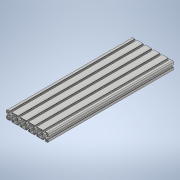
# Autodesk Inventor part: 20100 dai 300
Saved by Autodesk Inventor 2020 (Build 240168000, 168)
## iProperties
Created: 2020-04-28
Part Number: 20100 dai 300
Material: Generic
Document SubType Name: Modeling
Designer: Dell-T1700
Density: 1 g/cm^3
Appearance: Default
Author: Dell-T1700
Autodesk Inventor part; units mm, degrees
ref_plane "YZ Plane" through (0, 0, 0) normal (1, 0, 0) x (0, 1, 0)
ref_plane "XZ Plane" through (0, 0, 0) normal (0, 1, 0) x (-1, 0, 0)
ref_plane "XY Plane" through (0, 0, 0) normal (0, 0, 1) x (1, 0, 0)
sketch "Sketch1" plane through (0, 0, 0) normal (0, 0, 1) x (1, 0, 0)
  line L0 (-2.55, -10) -> (-2.55, -9.25)
  line L1 (-2.55, -9.25) -> (-2.05, -9.25)
  line L2 (-7.75, -10) -> (-2.55, -10)
  line L3 (-2.05, -9.25) -> (-2.05, -7)
  line L4 (-2.05, -7) -> (-3.05, -7)
  line L5 (-3.05, -9.1) -> (-3.05, -7)
  line L6 (-3.05, -9.1) -> (-5.125, -9.1)
  line L7 (-5.125, -9.1) -> (-5.125, -5.8321)
  line L8 (-8, -9.25) -> (-5.775, -9.25)
  line L9 (-5.775, -9.25) -> (-5.775, -5.775)
  line L10 (-2.2929, -3) -> (2.2929, -3)
  line L11 (3, -2.2929) -> (3, 2.2929)
  line L12 (2.2929, 3) -> (-2.2929, 3)
  line L13 (-3, 2.2929) -> (-3, -2.2929)
  line L14 (-2.2929, -3) -> (-5.125, -5.8321)
  line L15 (-3, -2.2929) -> (-5.8321, -5.125)
  line L16 (-9.1, -5.125) -> (-5.8321, -5.125)
  line L17 (-9.25, -5.775) -> (-5.775, -5.775)
  line L18 (-9.25, -8) -> (-9.25, -5.775)
  line L19 (-10, -7.75) -> (-10, -2.55)
  line L20 (-9.1, -3.05) -> (-9.1, -5.125)
  line L21 (-9.1, -3.05) -> (-7, -3.05)
  line L22 (-9.25, -2.55) -> (-9.25, -2.05)
  line L23 (-9.25, -2.05) -> (-7, -2.05)
  line L24 (-7, -2.05) -> (-7, -3.05)
  line L25 (-10, -2.55) -> (-9.25, -2.55)
  arc A0 (-9.25, -8) -> (-8, -9.25) centre (-8, -8) ccw
  arc A1 (-10, -7.75) -> (-7.75, -10) centre (-7.75, -7.75) ccw
  line L26 (3, -2.2929) -> (5.8321, -5.125)
  line L27 (2.2929, -3) -> (5.125, -5.8321)
  line L28 (5.775, -9.25) -> (5.775, -5.775)
  line L29 (8, -9.25) -> (5.775, -9.25)
  line L30 (7.75, -10) -> (2.55, -10)
  line L31 (3.05, -9.1) -> (5.125, -9.1)
  line L32 (2.55, -10) -> (2.55, -9.25)
  line L33 (3.05, -9.1) -> (3.05, -7)
  line L34 (2.05, -9.25) -> (2.05, -7)
  line L35 (2.55, -9.25) -> (2.05, -9.25)
  line L36 (2.05, -7) -> (3.05, -7)
  line L37 (5.125, -9.1) -> (5.125, -5.8321)
  arc A2 (8, -9.25) -> (9.25, -8) centre (8, -8) ccw
  arc A3 (7.75, -10) -> (10, -7.75) centre (7.75, -7.75) ccw
  line L38 (9.25, -8) -> (9.25, -5.775)
  line L39 (10, -7.75) -> (10, -2.55)
  line L40 (9.25, -5.775) -> (5.775, -5.775)
  line L41 (9.1, -5.125) -> (5.8321, -5.125)
  line L42 (9.1, -3.05) -> (7, -3.05)
  line L43 (7, -2.05) -> (7, -3.05)
  line L44 (9.25, -2.05) -> (7, -2.05)
  line L45 (9.25, -2.55) -> (9.25, -2.05)
  line L46 (10, -2.55) -> (9.25, -2.55)
  line L47 (9.1, -3.05) -> (9.1, -5.125)
  line L48 (2.2929, 3) -> (5.125, 5.8321)
  line L49 (3, 2.2929) -> (5.8321, 5.125)
  line L50 (9.25, 5.775) -> (5.775, 5.775)
  line L51 (9.25, 8) -> (9.25, 5.775)
  line L52 (10, 7.75) -> (10, 2.55)
  line L53 (9.1, 3.05) -> (9.1, 5.125)
  line L54 (10, 2.55) -> (9.25, 2.55)
  line L55 (9.1, 3.05) -> (7, 3.05)
  line L56 (9.25, 2.05) -> (7, 2.05)
  line L57 (9.25, 2.55) -> (9.25, 2.05)
  line L58 (7, 2.05) -> (7, 3.05)
  line L59 (9.1, 5.125) -> (5.8321, 5.125)
  arc A4 (9.25, 8) -> (8, 9.25) centre (8, 8) ccw
  arc A5 (10, 7.75) -> (7.75, 10) centre (7.75, 7.75) ccw
  line L60 (8, 9.25) -> (5.775, 9.25)
  line L61 (7.75, 10) -> (2.55, 10)
  line L62 (5.775, 9.25) -> (5.775, 5.775)
  line L63 (5.125, 9.1) -> (5.125, 5.8321)
  line L64 (3.05, 9.1) -> (3.05, 7)
  line L65 (2.05, 7) -> (3.05, 7)
  line L66 (2.05, 9.25) -> (2.05, 7)
  line L67 (2.55, 9.25) -> (2.05, 9.25)
  line L68 (2.55, 10) -> (2.55, 9.25)
  line L69 (3.05, 9.1) -> (5.125, 9.1)
  line L70 (-3, 2.2929) -> (-5.8321, 5.125)
  line L71 (-2.2929, 3) -> (-5.125, 5.8321)
  line L72 (-5.775, 9.25) -> (-5.775, 5.775)
  line L73 (-8, 9.25) -> (-5.775, 9.25)
  line L74 (-7.75, 10) -> (-2.55, 10)
  line L75 (-3.05, 9.1) -> (-5.125, 9.1)
  line L76 (-2.55, 10) -> (-2.55, 9.25)
  line L77 (-3.05, 9.1) -> (-3.05, 7)
  line L78 (-2.05, 9.25) -> (-2.05, 7)
  line L79 (-2.55, 9.25) -> (-2.05, 9.25)
  line L80 (-2.05, 7) -> (-3.05, 7)
  line L81 (-5.125, 9.1) -> (-5.125, 5.8321)
  arc A6 (-8, 9.25) -> (-9.25, 8) centre (-8, 8) ccw
  arc A7 (-7.75, 10) -> (-10, 7.75) centre (-7.75, 7.75) ccw
  line L82 (-9.25, 8) -> (-9.25, 5.775)
  line L83 (-10, 7.75) -> (-10, 2.55)
  line L84 (-9.25, 5.775) -> (-5.775, 5.775)
  line L85 (-9.1, 5.125) -> (-5.8321, 5.125)
  line L86 (-9.1, 3.05) -> (-7, 3.05)
  line L87 (-7, 2.05) -> (-7, 3.05)
  line L88 (-9.25, 2.05) -> (-7, 2.05)
  line L89 (-9.25, 2.55) -> (-9.25, 2.05)
  line L90 (-10, 2.55) -> (-9.25, 2.55)
  line L91 (-9.1, 3.05) -> (-9.1, 5.125)
  circle A8 centre (0, 0) radius 2
  line L92 (17.45, -10) -> (17.45, -9.25)
  line L93 (17.45, -9.25) -> (17.95, -9.25)
  line L94 (12.25, -10) -> (17.45, -10)
  line L95 (17.95, -9.25) -> (17.95, -7)
  line L96 (17.95, -7) -> (16.95, -7)
  line L97 (17, -2.2929) -> (14.1679, -5.125)
  line L98 (17.7071, -3) -> (14.875, -5.8321)
  line L99 (14.225, -9.25) -> (14.225, -5.775)
  line L100 (14.875, -9.1) -> (14.875, -5.8321)
  line L101 (16.95, -9.1) -> (16.95, -7)
  line L102 (16.95, -9.1) -> (14.875, -9.1)
  line L103 (12, -9.25) -> (14.225, -9.25)
  line L104 (10.75, -5.775) -> (14.225, -5.775)
  line L105 (10.9, -5.125) -> (14.1679, -5.125)
  line L106 (10.75, -8) -> (10.75, -5.775)
  line L107 (10, -7.75) -> (10, -2.55)
  line L108 (10.9, -3.05) -> (10.9, -5.125)
  line L109 (13, -2.05) -> (13, -3.05)
  line L110 (10.9, -3.05) -> (13, -3.05)
  line L111 (10.75, -2.05) -> (13, -2.05)
  line L112 (10.75, -2.55) -> (10.75, -2.05)
  line L113 (10, -2.55) -> (10.75, -2.55)
  arc A9 (10, -7.75) -> (12.25, -10) centre (12.25, -7.75) ccw
  arc A10 (10.75, -8) -> (12, -9.25) centre (12, -8) ccw
  line L114 (23, -2.2929) -> (25.8321, -5.125)
  line L115 (22.2929, -3) -> (25.125, -5.8321)
  line L116 (22.05, -9.25) -> (22.05, -7)
  line L117 (22.55, -10) -> (22.55, -9.25)
  line L118 (22.55, -9.25) -> (22.05, -9.25)
  line L119 (22.05, -7) -> (23.05, -7)
  line L120 (23.05, -9.1) -> (23.05, -7)
  line L121 (23.05, -9.1) -> (25.125, -9.1)
  line L122 (27.75, -10) -> (22.55, -10)
  line L123 (27, -2.05) -> (27, -3.05)
  line L124 (25.125, -9.1) -> (25.125, -5.8321)
  line L125 (29.1, -5.125) -> (25.8321, -5.125)
  line L126 (29.1, -3.05) -> (27, -3.05)
  line L127 (29.1, -3.05) -> (29.1, -5.125)
  line L128 (29.25, -2.05) -> (27, -2.05)
  line L129 (29.25, -2.55) -> (29.25, -2.05)
  line L130 (30, -2.55) -> (29.25, -2.55)
  line L131 (30, -7.75) -> (30, -2.55)
  line L132 (25.775, -9.25) -> (25.775, -5.775)
  line L133 (29.25, -5.775) -> (25.775, -5.775)
  line L134 (28, -9.25) -> (25.775, -9.25)
  line L135 (29.25, -8) -> (29.25, -5.775)
  arc A11 (28, -9.25) -> (29.25, -8) centre (28, -8) ccw
  arc A12 (27.75, -10) -> (30, -7.75) centre (27.75, -7.75) ccw
  arc A13 (29.25, 8) -> (28, 9.25) centre (28, 8) ccw
  arc A14 (30, 7.75) -> (27.75, 10) centre (27.75, 7.75) ccw
  line L136 (29.25, 2.05) -> (27, 2.05)
  line L137 (29.25, 2.55) -> (29.25, 2.05)
  line L138 (30, 2.55) -> (29.25, 2.55)
  line L139 (27, 2.05) -> (27, 3.05)
  line L140 (29.1, 3.05) -> (27, 3.05)
  line L141 (29.1, 3.05) -> (29.1, 5.125)
  line L142 (29.1, 5.125) -> (25.8321, 5.125)
  line L143 (23, 2.2929) -> (25.8321, 5.125)
  line L144 (22.2929, 3) -> (25.125, 5.8321)
  line L145 (30, 7.75) -> (30, 2.55)
  line L146 (29.25, 5.775) -> (25.775, 5.775)
  line L147 (29.25, 8) -> (29.25, 5.775)
  line L148 (28, 9.25) -> (25.775, 9.25)
  line L149 (25.775, 9.25) -> (25.775, 5.775)
  line L150 (25.125, 9.1) -> (25.125, 5.8321)
  line L151 (27.75, 10) -> (22.55, 10)
  line L152 (23.05, 9.1) -> (25.125, 9.1)
  line L153 (22.55, 10) -> (22.55, 9.25)
  line L154 (23.05, 9.1) -> (23.05, 7)
  line L155 (22.05, 7) -> (23.05, 7)
  line L156 (22.05, 9.25) -> (22.05, 7)
  line L157 (22.55, 9.25) -> (22.05, 9.25)
  line L158 (17.95, 9.25) -> (17.95, 7)
  line L159 (17.45, 9.25) -> (17.95, 9.25)
  line L160 (17.95, 7) -> (16.95, 7)
  line L161 (16.95, 9.1) -> (16.95, 7)
  line L162 (14.225, 9.25) -> (14.225, 5.775)
  line L163 (12, 9.25) -> (14.225, 9.25)
  line L164 (10.9, 5.125) -> (14.1679, 5.125)
  line L165 (10.75, 5.775) -> (14.225, 5.775)
  line L166 (10.75, 8) -> (10.75, 5.775)
  arc A15 (12, 9.25) -> (10.75, 8) centre (12, 8) ccw
  arc A16 (12.25, 10) -> (10, 7.75) centre (12.25, 7.75) ccw
  line L167 (10, 7.75) -> (10, 2.55)
  line L168 (10.9, 3.05) -> (10.9, 5.125)
  line L169 (13, 2.05) -> (13, 3.05)
  line L170 (10.9, 3.05) -> (13, 3.05)
  line L171 (10.75, 2.05) -> (13, 2.05)
  line L172 (10.75, 2.55) -> (10.75, 2.05)
  line L173 (10, 2.55) -> (10.75, 2.55)
  line L174 (17.7071, -3) -> (22.2929, -3)
  line L175 (23, -2.2929) -> (23, 2.2929)
  line L176 (22.2929, 3) -> (17.7071, 3)
  line L177 (17, 2.2929) -> (17, -2.2929)
  line L178 (17.45, 10) -> (17.45, 9.25)
  circle A17 centre (20, 0) radius 2
  line L179 (16.95, 9.1) -> (14.875, 9.1)
  line L180 (14.875, 9.1) -> (14.875, 5.8321)
  line L181 (17.7071, 3) -> (14.875, 5.8321)
  line L182 (17, 2.2929) -> (14.1679, 5.125)
  line L183 (12.25, 10) -> (17.45, 10)
  line L184 (37.45, -10) -> (37.45, -9.25)
  line L185 (37.45, -9.25) -> (37.95, -9.25)
  line L186 (32.25, -10) -> (37.45, -10)
  line L187 (37.95, -9.25) -> (37.95, -7)
  line L188 (37.95, -7) -> (36.95, -7)
  line L189 (37, -2.2929) -> (34.1679, -5.125)
  line L190 (37.7071, -3) -> (34.875, -5.8321)
  line L191 (34.225, -9.25) -> (34.225, -5.775)
  line L192 (34.875, -9.1) -> (34.875, -5.8321)
  line L193 (36.95, -9.1) -> (36.95, -7)
  line L194 (36.95, -9.1) -> (34.875, -9.1)
  line L195 (32, -9.25) -> (34.225, -9.25)
  line L196 (30.75, -5.775) -> (34.225, -5.775)
  line L197 (30.9, -5.125) -> (34.1679, -5.125)
  line L198 (30.75, -8) -> (30.75, -5.775)
  line L199 (30, -7.75) -> (30, -2.55)
  line L200 (30.9, -3.05) -> (30.9, -5.125)
  line L201 (33, -2.05) -> (33, -3.05)
  line L202 (30.9, -3.05) -> (33, -3.05)
  line L203 (30.75, -2.05) -> (33, -2.05)
  line L204 (30.75, -2.55) -> (30.75, -2.05)
  line L205 (30, -2.55) -> (30.75, -2.55)
  arc A18 (30, -7.75) -> (32.25, -10) centre (32.25, -7.75) ccw
  arc A19 (30.75, -8) -> (32, -9.25) centre (32, -8) ccw
  line L206 (43, -2.2929) -> (45.8321, -5.125)
  line L207 (42.2929, -3) -> (45.125, -5.8321)
  line L208 (42.05, -9.25) -> (42.05, -7)
  line L209 (42.55, -10) -> (42.55, -9.25)
  line L210 (42.55, -9.25) -> (42.05, -9.25)
  line L211 (42.05, -7) -> (43.05, -7)
  line L212 (43.05, -9.1) -> (43.05, -7)
  line L213 (43.05, -9.1) -> (45.125, -9.1)
  line L214 (47.75, -10) -> (42.55, -10)
  line L215 (47, -2.05) -> (47, -3.05)
  line L216 (45.125, -9.1) -> (45.125, -5.8321)
  line L217 (49.1, -5.125) -> (45.8321, -5.125)
  line L218 (49.1, -3.05) -> (47, -3.05)
  line L219 (49.1, -3.05) -> (49.1, -5.125)
  line L220 (49.25, -2.05) -> (47, -2.05)
  line L221 (49.25, -2.55) -> (49.25, -2.05)
  line L222 (50, -2.55) -> (49.25, -2.55)
  line L223 (50, -7.75) -> (50, -2.55)
  line L224 (45.775, -9.25) -> (45.775, -5.775)
  line L225 (49.25, -5.775) -> (45.775, -5.775)
  line L226 (48, -9.25) -> (45.775, -9.25)
  line L227 (49.25, -8) -> (49.25, -5.775)
  arc A20 (48, -9.25) -> (49.25, -8) centre (48, -8) ccw
  arc A21 (47.75, -10) -> (50, -7.75) centre (47.75, -7.75) ccw
  arc A22 (49.25, 8) -> (48, 9.25) centre (48, 8) ccw
  arc A23 (50, 7.75) -> (47.75, 10) centre (47.75, 7.75) ccw
  line L228 (49.25, 2.05) -> (47, 2.05)
  line L229 (49.25, 2.55) -> (49.25, 2.05)
  line L230 (50, 2.55) -> (49.25, 2.55)
  line L231 (47, 2.05) -> (47, 3.05)
  line L232 (49.1, 3.05) -> (47, 3.05)
  line L233 (49.1, 3.05) -> (49.1, 5.125)
  line L234 (49.1, 5.125) -> (45.8321, 5.125)
  line L235 (43, 2.2929) -> (45.8321, 5.125)
  line L236 (42.2929, 3) -> (45.125, 5.8321)
  line L237 (50, 7.75) -> (50, 2.55)
  line L238 (49.25, 5.775) -> (45.775, 5.775)
  line L239 (49.25, 8) -> (49.25, 5.775)
  line L240 (48, 9.25) -> (45.775, 9.25)
  line L241 (45.775, 9.25) -> (45.775, 5.775)
  line L242 (45.125, 9.1) -> (45.125, 5.8321)
  line L243 (47.75, 10) -> (42.55, 10)
  line L244 (43.05, 9.1) -> (45.125, 9.1)
  line L245 (42.55, 10) -> (42.55, 9.25)
  line L246 (43.05, 9.1) -> (43.05, 7)
  line L247 (42.05, 7) -> (43.05, 7)
  line L248 (42.05, 9.25) -> (42.05, 7)
  line L249 (42.55, 9.25) -> (42.05, 9.25)
  line L250 (37.95, 9.25) -> (37.95, 7)
  line L251 (37.45, 9.25) -> (37.95, 9.25)
  line L252 (37.95, 7) -> (36.95, 7)
  line L253 (36.95, 9.1) -> (36.95, 7)
  line L254 (34.225, 9.25) -> (34.225, 5.775)
  line L255 (32, 9.25) -> (34.225, 9.25)
  line L256 (30.9, 5.125) -> (34.1679, 5.125)
  line L257 (30.75, 5.775) -> (34.225, 5.775)
  line L258 (30.75, 8) -> (30.75, 5.775)
  arc A24 (32, 9.25) -> (30.75, 8) centre (32, 8) ccw
  arc A25 (32.25, 10) -> (30, 7.75) centre (32.25, 7.75) ccw
  line L259 (30, 7.75) -> (30, 2.55)
  line L260 (30.9, 3.05) -> (30.9, 5.125)
  line L261 (33, 2.05) -> (33, 3.05)
  line L262 (30.9, 3.05) -> (33, 3.05)
  line L263 (30.75, 2.05) -> (33, 2.05)
  line L264 (30.75, 2.55) -> (30.75, 2.05)
  line L265 (30, 2.55) -> (30.75, 2.55)
  line L266 (37.7071, -3) -> (42.2929, -3)
  line L267 (43, -2.2929) -> (43, 2.2929)
  line L268 (42.2929, 3) -> (37.7071, 3)
  line L269 (37, 2.2929) -> (37, -2.2929)
  line L270 (37.45, 10) -> (37.45, 9.25)
  circle A26 centre (40, 0) radius 2
  line L271 (36.95, 9.1) -> (34.875, 9.1)
  line L272 (34.875, 9.1) -> (34.875, 5.8321)
  line L273 (37.7071, 3) -> (34.875, 5.8321)
  line L274 (37, 2.2929) -> (34.1679, 5.125)
  line L275 (32.25, 10) -> (37.45, 10)
  line L276 (57.45, -10) -> (57.45, -9.25)
  line L277 (57.45, -9.25) -> (57.95, -9.25)
  line L278 (52.25, -10) -> (57.45, -10)
  line L279 (57.95, -9.25) -> (57.95, -7)
  line L280 (57.95, -7) -> (56.95, -7)
  line L281 (57, -2.2929) -> (54.1679, -5.125)
  line L282 (57.7071, -3) -> (54.875, -5.8321)
  line L283 (54.225, -9.25) -> (54.225, -5.775)
  line L284 (54.875, -9.1) -> (54.875, -5.8321)
  line L285 (56.95, -9.1) -> (56.95, -7)
  line L286 (56.95, -9.1) -> (54.875, -9.1)
  line L287 (52, -9.25) -> (54.225, -9.25)
  line L288 (50.75, -5.775) -> (54.225, -5.775)
  line L289 (50.9, -5.125) -> (54.1679, -5.125)
  line L290 (50.75, -8) -> (50.75, -5.775)
  line L291 (50, -7.75) -> (50, -2.55)
  line L292 (50.9, -3.05) -> (50.9, -5.125)
  line L293 (53, -2.05) -> (53, -3.05)
  line L294 (50.9, -3.05) -> (53, -3.05)
  line L295 (50.75, -2.05) -> (53, -2.05)
  line L296 (50.75, -2.55) -> (50.75, -2.05)
  line L297 (50, -2.55) -> (50.75, -2.55)
  arc A27 (50, -7.75) -> (52.25, -10) centre (52.25, -7.75) ccw
  arc A28 (50.75, -8) -> (52, -9.25) centre (52, -8) ccw
  line L298 (63, -2.2929) -> (65.8321, -5.125)
  line L299 (62.2929, -3) -> (65.125, -5.8321)
  line L300 (62.05, -9.25) -> (62.05, -7)
  line L301 (62.55, -10) -> (62.55, -9.25)
  line L302 (62.55, -9.25) -> (62.05, -9.25)
  line L303 (62.05, -7) -> (63.05, -7)
  line L304 (63.05, -9.1) -> (63.05, -7)
  line L305 (63.05, -9.1) -> (65.125, -9.1)
  line L306 (67.75, -10) -> (62.55, -10)
  line L307 (67, -2.05) -> (67, -3.05)
  line L308 (65.125, -9.1) -> (65.125, -5.8321)
  line L309 (69.1, -5.125) -> (65.8321, -5.125)
  line L310 (69.1, -3.05) -> (67, -3.05)
  line L311 (69.1, -3.05) -> (69.1, -5.125)
  line L312 (69.25, -2.05) -> (67, -2.05)
  line L313 (69.25, -2.55) -> (69.25, -2.05)
  line L314 (70, -2.55) -> (69.25, -2.55)
  line L315 (70, -7.75) -> (70, -2.55)
  line L316 (65.775, -9.25) -> (65.775, -5.775)
  line L317 (69.25, -5.775) -> (65.775, -5.775)
  line L318 (68, -9.25) -> (65.775, -9.25)
  line L319 (69.25, -8) -> (69.25, -5.775)
  arc A29 (68, -9.25) -> (69.25, -8) centre (68, -8) ccw
  arc A30 (67.75, -10) -> (70, -7.75) centre (67.75, -7.75) ccw
  arc A31 (69.25, 8) -> (68, 9.25) centre (68, 8) ccw
  arc A32 (70, 7.75) -> (67.75, 10) centre (67.75, 7.75) ccw
  line L320 (69.25, 2.05) -> (67, 2.05)
  line L321 (69.25, 2.55) -> (69.25, 2.05)
  line L322 (70, 2.55) -> (69.25, 2.55)
  line L323 (67, 2.05) -> (67, 3.05)
  line L324 (69.1, 3.05) -> (67, 3.05)
  line L325 (69.1, 3.05) -> (69.1, 5.125)
  line L326 (69.1, 5.125) -> (65.8321, 5.125)
  line L327 (63, 2.2929) -> (65.8321, 5.125)
  line L328 (62.2929, 3) -> (65.125, 5.8321)
  line L329 (70, 7.75) -> (70, 2.55)
  line L330 (69.25, 5.775) -> (65.775, 5.775)
  line L331 (69.25, 8) -> (69.25, 5.775)
  line L332 (68, 9.25) -> (65.775, 9.25)
  line L333 (65.775, 9.25) -> (65.775, 5.775)
  line L334 (65.125, 9.1) -> (65.125, 5.8321)
  line L335 (67.75, 10) -> (62.55, 10)
  line L336 (63.05, 9.1) -> (65.125, 9.1)
  line L337 (62.55, 10) -> (62.55, 9.25)
  line L338 (63.05, 9.1) -> (63.05, 7)
  line L339 (62.05, 7) -> (63.05, 7)
  line L340 (62.05, 9.25) -> (62.05, 7)
  line L341 (62.55, 9.25) -> (62.05, 9.25)
  line L342 (57.95, 9.25) -> (57.95, 7)
  line L343 (57.45, 9.25) -> (57.95, 9.25)
  line L344 (57.95, 7) -> (56.95, 7)
  line L345 (56.95, 9.1) -> (56.95, 7)
  line L346 (54.225, 9.25) -> (54.225, 5.775)
  line L347 (52, 9.25) -> (54.225, 9.25)
  line L348 (50.9, 5.125) -> (54.1679, 5.125)
  line L349 (50.75, 5.775) -> (54.225, 5.775)
  line L350 (50.75, 8) -> (50.75, 5.775)
  arc A33 (52, 9.25) -> (50.75, 8) centre (52, 8) ccw
  arc A34 (52.25, 10) -> (50, 7.75) centre (52.25, 7.75) ccw
  line L351 (50, 7.75) -> (50, 2.55)
  line L352 (50.9, 3.05) -> (50.9, 5.125)
  line L353 (53, 2.05) -> (53, 3.05)
  line L354 (50.9, 3.05) -> (53, 3.05)
  line L355 (50.75, 2.05) -> (53, 2.05)
  line L356 (50.75, 2.55) -> (50.75, 2.05)
  line L357 (50, 2.55) -> (50.75, 2.55)
  line L358 (57.7071, -3) -> (62.2929, -3)
  line L359 (63, -2.2929) -> (63, 2.2929)
  line L360 (62.2929, 3) -> (57.7071, 3)
  line L361 (57, 2.2929) -> (57, -2.2929)
  line L362 (57.45, 10) -> (57.45, 9.25)
  circle A35 centre (60, 0) radius 2
  line L363 (56.95, 9.1) -> (54.875, 9.1)
  line L364 (54.875, 9.1) -> (54.875, 5.8321)
  line L365 (57.7071, 3) -> (54.875, 5.8321)
  line L366 (57, 2.2929) -> (54.1679, 5.125)
  line L367 (52.25, 10) -> (57.45, 10)
  line L368 (77.45, -10) -> (77.45, -9.25)
  line L369 (77.45, -9.25) -> (77.95, -9.25)
  line L370 (72.25, -10) -> (77.45, -10)
  line L371 (77.95, -9.25) -> (77.95, -7)
  line L372 (77.95, -7) -> (76.95, -7)
  line L373 (77, -2.2929) -> (74.1679, -5.125)
  line L374 (77.7071, -3) -> (74.875, -5.8321)
  line L375 (74.225, -9.25) -> (74.225, -5.775)
  line L376 (74.875, -9.1) -> (74.875, -5.8321)
  line L377 (76.95, -9.1) -> (76.95, -7)
  line L378 (76.95, -9.1) -> (74.875, -9.1)
  line L379 (72, -9.25) -> (74.225, -9.25)
  line L380 (70.75, -5.775) -> (74.225, -5.775)
  line L381 (70.9, -5.125) -> (74.1679, -5.125)
  line L382 (70.75, -8) -> (70.75, -5.775)
  line L383 (70, -7.75) -> (70, -2.55)
  line L384 (70.9, -3.05) -> (70.9, -5.125)
  line L385 (73, -2.05) -> (73, -3.05)
  line L386 (70.9, -3.05) -> (73, -3.05)
  line L387 (70.75, -2.05) -> (73, -2.05)
  line L388 (70.75, -2.55) -> (70.75, -2.05)
  line L389 (70, -2.55) -> (70.75, -2.55)
  arc A36 (70, -7.75) -> (72.25, -10) centre (72.25, -7.75) ccw
  arc A37 (70.75, -8) -> (72, -9.25) centre (72, -8) ccw
  line L390 (83, -2.2929) -> (85.8321, -5.125)
  line L391 (82.2929, -3) -> (85.125, -5.8321)
  line L392 (82.05, -9.25) -> (82.05, -7)
  line L393 (82.55, -10) -> (82.55, -9.25)
  line L394 (82.55, -9.25) -> (82.05, -9.25)
  line L395 (82.05, -7) -> (83.05, -7)
  line L396 (83.05, -9.1) -> (83.05, -7)
  line L397 (83.05, -9.1) -> (85.125, -9.1)
  line L398 (87.75, -10) -> (82.55, -10)
  line L399 (87, -2.05) -> (87, -3.05)
  line L400 (85.125, -9.1) -> (85.125, -5.8321)
  line L401 (89.1, -5.125) -> (85.8321, -5.125)
  line L402 (89.1, -3.05) -> (87, -3.05)
  line L403 (89.1, -3.05) -> (89.1, -5.125)
  line L404 (89.25, -2.05) -> (87, -2.05)
  line L405 (89.25, -2.55) -> (89.25, -2.05)
  line L406 (90, -2.55) -> (89.25, -2.55)
  line L407 (90, -7.75) -> (90, -2.55)
  line L408 (85.775, -9.25) -> (85.775, -5.775)
  line L409 (89.25, -5.775) -> (85.775, -5.775)
  line L410 (88, -9.25) -> (85.775, -9.25)
  line L411 (89.25, -8) -> (89.25, -5.775)
  arc A38 (88, -9.25) -> (89.25, -8) centre (88, -8) ccw
  arc A39 (87.75, -10) -> (90, -7.75) centre (87.75, -7.75) ccw
  arc A40 (89.25, 8) -> (88, 9.25) centre (88, 8) ccw
  arc A41 (90, 7.75) -> (87.75, 10) centre (87.75, 7.75) ccw
  line L412 (89.25, 2.05) -> (87, 2.05)
  line L413 (89.25, 2.55) -> (89.25, 2.05)
  line L414 (90, 2.55) -> (89.25, 2.55)
  line L415 (87, 2.05) -> (87, 3.05)
  line L416 (89.1, 3.05) -> (87, 3.05)
  line L417 (89.1, 3.05) -> (89.1, 5.125)
  line L418 (89.1, 5.125) -> (85.8321, 5.125)
  line L419 (83, 2.2929) -> (85.8321, 5.125)
  line L420 (82.2929, 3) -> (85.125, 5.8321)
  line L421 (90, 7.75) -> (90, 2.55)
  line L422 (89.25, 5.775) -> (85.775, 5.775)
  line L423 (89.25, 8) -> (89.25, 5.775)
  line L424 (88, 9.25) -> (85.775, 9.25)
  line L425 (85.775, 9.25) -> (85.775, 5.775)
  line L426 (85.125, 9.1) -> (85.125, 5.8321)
  line L427 (87.75, 10) -> (82.55, 10)
  line L428 (83.05, 9.1) -> (85.125, 9.1)
  line L429 (82.55, 10) -> (82.55, 9.25)
  line L430 (83.05, 9.1) -> (83.05, 7)
  line L431 (82.05, 7) -> (83.05, 7)
  line L432 (82.05, 9.25) -> (82.05, 7)
  line L433 (82.55, 9.25) -> (82.05, 9.25)
  line L434 (77.95, 9.25) -> (77.95, 7)
  line L435 (77.45, 9.25) -> (77.95, 9.25)
  line L436 (77.95, 7) -> (76.95, 7)
  line L437 (76.95, 9.1) -> (76.95, 7)
  line L438 (74.225, 9.25) -> (74.225, 5.775)
  line L439 (72, 9.25) -> (74.225, 9.25)
  line L440 (70.9, 5.125) -> (74.1679, 5.125)
  line L441 (70.75, 5.775) -> (74.225, 5.775)
  line L442 (70.75, 8) -> (70.75, 5.775)
  arc A42 (72, 9.25) -> (70.75, 8) centre (72, 8) ccw
  arc A43 (72.25, 10) -> (70, 7.75) centre (72.25, 7.75) ccw
  line L443 (70, 7.75) -> (70, 2.55)
  line L444 (70.9, 3.05) -> (70.9, 5.125)
  line L445 (73, 2.05) -> (73, 3.05)
  line L446 (70.9, 3.05) -> (73, 3.05)
  line L447 (70.75, 2.05) -> (73, 2.05)
  line L448 (70.75, 2.55) -> (70.75, 2.05)
  line L449 (70, 2.55) -> (70.75, 2.55)
  line L450 (77.7071, -3) -> (82.2929, -3)
  line L451 (83, -2.2929) -> (83, 2.2929)
  line L452 (82.2929, 3) -> (77.7071, 3)
  line L453 (77, 2.2929) -> (77, -2.2929)
  line L454 (77.45, 10) -> (77.45, 9.25)
  circle A44 centre (80, 0) radius 2
  line L455 (76.95, 9.1) -> (74.875, 9.1)
  line L456 (74.875, 9.1) -> (74.875, 5.8321)
  line L457 (77.7071, 3) -> (74.875, 5.8321)
  line L458 (77, 2.2929) -> (74.1679, 5.125)
  line L459 (72.25, 10) -> (77.45, 10)
  line L460 (7.75, 10) -> (12.25, 10)
  line L461 (7.75, -10) -> (12.25, -10)
  line L462 (27.75, -10) -> (32.25, -10)
  line L463 (47.75, -10) -> (52.25, -10)
  line L464 (67.75, -10) -> (72.25, -10)
  line L465 (32.25, 10) -> (27.75, 10)
  line L466 (47.75, 10) -> (52.25, 10)
  line L467 (67.75, 10) -> (72.25, 10)
  line L468 (5.775, 5.775) -> (5.775, 5.0679)
  line L469 (14.225, 5.775) -> (14.225, 5.0679)
  line L470 (8, 9.25) -> (14.225, 9.25)
  line L471 (8, -9.25) -> (12, -9.25)
  line L472 (5.775, -5.775) -> (5.775, -5.0679)
  line L473 (14.225, -5.775) -> (14.225, -5.0679)
  line L474 (25.775, -5.775) -> (25.775, -5.0679)
  line L475 (32, 9.25) -> (28, 9.25)
  line L476 (25.775, 5.775) -> (25.775, 5.0679)
  line L477 (32, -9.25) -> (28, -9.25)
  line L478 (34.225, -5.775) -> (34.225, -5.0679)
  line L479 (45.775, -5.775) -> (45.775, -5.0679)
  line L480 (48, -9.25) -> (52, -9.25)
  line L481 (45.775, 5.775) -> (45.775, 5.0679)
  line L482 (54.225, 5.775) -> (54.225, 5.0679)
  line L483 (54.225, -5.775) -> (54.225, -5.0679)
  line L484 (65.775, -5.775) -> (65.775, -5.0679)
  line L485 (72, -9.25) -> (68, -9.25)
  line L486 (68, 9.25) -> (72, 9.25)
  line L487 (65.775, 5.775) -> (65.775, 5.0679)
  line L488 (74.225, 5.775) -> (74.225, 5.0679)
  line L489 (74.225, -5.775) -> (74.225, -5.0679)
  line L490 (48, 9.25) -> (52, 9.25)
  line L491 (34.225, 5.775) -> (34.225, 5.0679)
  point P0 (-10, -10)
  point P1 (10, -10)
  point P2 (10, 10)
  point P3 (-10, 10)
  point P4 (10, -10)
  point P5 (30, -10)
  point P6 (30, 10)
  point P7 (10, 10)
  point P8 (30, -10)
  point P9 (50, -10)
  point P10 (50, 10)
  point P11 (30, 10)
  point P12 (50, -10)
  point P13 (70, -10)
  point P14 (70, 10)
  point P15 (50, 10)
  point P16 (70, -10)
  point P17 (90, -10)
  point P18 (90, 10)
  point P19 (70, 10)
  point P20 (50.5729, 9.25)
  point P21 (49.4271, 9.25)
  dimension "d2" = 0.75
  dimension "d3" = 7.45
  dimension "d4" = 2.25
  dimension "d5" = 1
  dimension "d6" = 2.1
  dimension "d7" = 0.75
  dimension "d8" = 0.65
  dimension "d9" = 1.25
  dimension "d10" = 2.25
  dimension "d11" = 360
  dimension "d12" = 4
  dimension "d13" = 20
  dimension "d18" = 0.75
  dimension "d19" = 7.45
  dimension "d20" = 2.25
  dimension "d21" = 1
  dimension "d22" = 2.1
  dimension "d23" = 0.75
  dimension "d24" = 0.65
  dimension "d25" = 1.25
  dimension "d26" = 2.25
  dimension "d27" = 360
  dimension "d28" = 4
  dimension "d29" = 20
  dimension "d34" = 0.75
  dimension "d35" = 7.45
  dimension "d36" = 2.25
  dimension "d37" = 1
  dimension "d38" = 2.1
  dimension "d39" = 0.75
  dimension "d40" = 0.65
  dimension "d41" = 1.25
  dimension "d42" = 2.25
  dimension "d43" = 360
  dimension "d44" = 4
  dimension "d45" = 20
  dimension "d52" = 0.75
  dimension "d53" = 7.45
  dimension "d54" = 2.25
  dimension "d55" = 1
  dimension "d56" = 2.1
  dimension "d57" = 0.75
  dimension "d58" = 0.65
  dimension "d59" = 1.25
  dimension "d60" = 2.25
  dimension "d61" = 360
  dimension "d62" = 4
  dimension "d63" = 20
  dimension "d72" = 0.75
  dimension "d73" = 7.45
  dimension "d74" = 2.25
  dimension "d75" = 1
  dimension "d76" = 2.1
  dimension "d77" = 0.75
  dimension "d78" = 0.65
  dimension "d79" = 1.25
  dimension "d80" = 2.25
  dimension "d81" = 360
  dimension "d82" = 4
  dimension "d83" = 20
  constraints: 984 end point, 80 point on circle, 58 point on line, 45 centre point, 28 horizontal, 28 tangent, 18 perpendicular, 17 vertical, 16 parallel, 7 collinear, 5 coincident, 1045 other
  measures "d2" distance of L0.start L0.end
  measures "d3" distance of point (-10, -10) L0.start
  measures "d4" distance of L1.end L3.end
  measures "d5" distance of L3.end L4.end
  measures "d6" distance of L5.start L4.end
  measures "d7" distance between parallel lines of L2 L8
  measures "d8" distance between parallel lines of L7 L9
  measures "d9" radius of A0
  measures "d10" radius of A1
  measures "d12" diameter of A8
  measures "d13" distance between parallel lines of L83 L52
  measures "d18" distance of L92.start L92.end
  measures "d19" distance of point (10, -10) L92.start
  measures "d20" distance of L93.end L95.end
  measures "d21" distance of L95.end L96.end
  measures "d22" distance of L101.start L96.end
  measures "d23" distance between parallel lines of L94 L103
  measures "d24" distance between parallel lines of L100 L99
  measures "d25" radius of A10
  measures "d26" radius of A9
  measures "d28" diameter of A17
  measures "d29" distance between parallel lines of L167 L145
  measures "d34" distance of L184.start L184.end
  measures "d35" distance of point (30, -10) L184.start
  measures "d36" distance of L185.end L187.end
  measures "d37" distance of L187.end L188.end
  measures "d38" distance of L193.start L188.end
  measures "d39" distance between parallel lines of L186 L195
  measures "d40" distance between parallel lines of L192 L191
  measures "d41" radius of A19
  measures "d42" radius of A18
  measures "d44" diameter of A26
  measures "d45" distance between parallel lines of L259 L237
  measures "d52" distance of L276.start L276.end
  measures "d53" distance of point (50, -10) L276.start
  measures "d54" distance of L277.end L279.end
  measures "d55" distance of L279.end L280.end
  measures "d56" distance of L285.start L280.end
  measures "d57" distance between parallel lines of L278 L287
  measures "d58" distance between parallel lines of L284 L283
  measures "d59" radius of A28
  measures "d60" radius of A27
  measures "d62" diameter of A35
  measures "d63" distance between parallel lines of L351 L329
  measures "d72" distance of L368.start L368.end
  measures "d73" distance of point (70, -10) L368.start
  measures "d74" distance of L369.end L371.end
  measures "d75" distance of L371.end L372.end
  measures "d76" distance of L377.start L372.end
  measures "d77" distance between parallel lines of L370 L379
  measures "d78" distance between parallel lines of L376 L375
  measures "d79" radius of A37
  measures "d80" radius of A36
  measures "d82" diameter of A44
  measures "d83" distance between parallel lines of L443 L421
extrude "Extrusion2" add sketch "Sketch1" along normal blind 300 contours L2 A1 L19 L25 L22 L23 L24 L21 L20 L16 L15 L13 L70 L85 L91 L86 L87 L88 L89 L90 L83 A7 L74 L76 L79 L78 L80 L77 L75 L81 L71 L12 L48 L63 L69 L64 L65 L66 L67 L68 L61 A5 L470 L60 L62 L468 L49 L11 L26 L472 L28 L29 L471 A3 L30 L32 L35 L34 L36 L33 L31 L37 L27 L10 L14 L7 L6 L5 L4 L3 L1 L0 | A3 L471 A9 L461 | A9 L471 L103 L99 L473 L97 L177 L182 L469 L162 L163 L470 A16 L183 L178 L159 L158 L160 L161 L179 L180 L181 L176 L144 L150 L152 L154 L155 L156 L157 L153 L151 A14 L475 L148 L149 L476 L143 L175 L114 L474 L132 L134 L477 A12 L122 L117 L118 L116 L119 L120 L121 L124 L115 L174 L98 L100 L102 L101 L96 L95 L93 L92 L94 | A5 L460 A16 L470 | A12 L477 A18 L462 | A18 L477 L195 L191 L478 L189 L269 L274 L491 L254 L255 L475 A25 L275 L270 L251 L250 L252 L253 L271 L272 L273 L268 L236 L242 L244 L246 L247 L248 L249 L245 L243 A23 L490 L240 L241 L481 L235 L267 L206 L479 L224 L226 L480 A21 L214 L209 L210 L208 L211 L212 L213 L216 L207 L266 L190 L192 L194 L193 L188 L187 L185 L184 L186 | A14 L465 A25 L475 | A21 L480 A27 L463 | A27 L480 L287 L283 L483 L281 L361 L366 L482 L346 L347 L490 A34 L367 L362 L343 L342 L344 L345 L363 L364 L365 L360 L328 L334 L336 L338 L339 L340 L341 L337 L335 A32 L486 L332 L333 L487 L327 L359 L298 L484 L316 L318 L485 A30 L306 L301 L302 L300 L303 L304 L305 L308 L299 L358 L282 L284 L286 L285 L280 L279 L277 L276 L278 | A23 L466 A34 L490 | A30 L485 A36 L464 | A36 L485 L379 L375 L489 L373 L453 L458 L488 L438 L439 L486 A43 L459 L454 L435 L434 L436 L437 L455 L456 L457 L452 L420 L426 L428 L430 L431 L432 L433 L429 L427 A41 L421 L414 L413 L412 L415 L416 L417 L418 L419 L451 L390 L401 L403 L402 L399 L404 L405 L406 L407 A39 L398 L393 L394 L392 L395 L396 L397 L400 L391 L450 L374 L376 L378 L377 L372 L371 L369 L368 L370 | A32 L467 A43 L486
body "Solid2"
